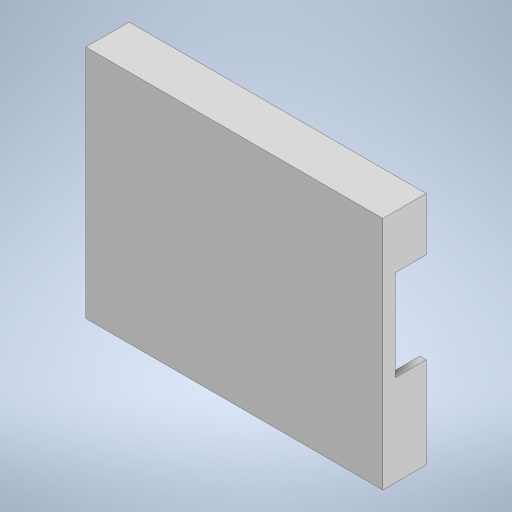
# Autodesk Inventor part: couvercle
Saved by Autodesk Inventor 2024 (Build 280153000, 153)
## iProperties
Created: 2024-03-05
Part Number: couvercle
Material: Générique
Document SubType Name: Modeling
Designer: phaly
Density: 1 g/cm^3
Appearance: Par défaut
Author: phaly
Autodesk Inventor part; units mm, degrees
ref_plane "YZ Plane" through (0, 0, 0) normal (1, 0, 0) x (0, 1, 0)
ref_plane "XZ Plane" through (0, 0, 0) normal (0, 1, 0) x (-1, 0, 0)
sketch "Esquisse1" plane through (0, 0, 0) normal (0, 0, 1) x (1, 0, 0)
  line L0 (-45.5759, 93.3928) -> (-189.5759, 93.3928) projected
  line L1 (-189.5759, 93.3928) -> (-189.5759, -20.6072) projected
  line L2 (-45.5759, -20.6072) -> (-45.5759, 93.3928) projected
  line L3 (-189.5759, -20.6072) -> (-45.5759, -20.6072) projected
  line L4 (-189.5759, 93.3928) -> (-45.5759, 93.3928)
  line L5 (-45.5759, 93.3928) -> (-45.5759, -20.6072)
  line L6 (-45.5759, -20.6072) -> (-189.5759, -20.6072)
  line L7 (-189.5759, -20.6072) -> (-189.5759, 93.3928)
  point P0 (0, 0)
  dimension "d20" = 114
  dimension "d21" = 144
  constraints: 8 end point, 2 parallel, 1 horizontal, 1 perpendicular
  measures "d20" distance of L0.end L1.end
  measures "d21" distance of L1.end L2.start
extrude "Extrusion1" add sketch "Esquisse1" along normal blind 21
sketch "Esquisse2" plane through (0, 0, 0) normal (0, 0, -1) x (-1, 0, 0)
  line L0 (186.5759, -17.6072) -> (48.5759, -17.6072)
  line L1 (48.5759, -17.6072) -> (48.5759, 90.3928)
  line L2 (48.5759, 90.3928) -> (186.5759, 90.3928)
  line L3 (186.5759, 90.3928) -> (186.5759, -17.6072)
  line L4 (189.5759, -20.6072) -> (45.5759, -20.6072) projected
  line L5 (45.5759, 93.3928) -> (189.5759, 93.3928) projected
  line L6 (189.5759, 93.3928) -> (189.5759, -20.6072) projected
  line L7 (45.5759, -20.6072) -> (45.5759, 93.3928) projected
  point P0 (0, 0)
  dimension "d2" = 3
  dimension "d4" = 3
  dimension "d5" = 3
  dimension "d6" = 3
  constraints: 8 end point, 2 parallel, 1 horizontal, 1 perpendicular
  measures "d2" distance between parallel lines of L4 L0
  measures "d4" distance between parallel lines of L6 L3
  measures "d5" distance between parallel lines of L5 L2
  measures "d6" distance between parallel lines of L7 L1
extrude "Extrusion3" cut sketch "Esquisse2" against normal blind 17 contours L0 L1 L2 L3
ref_plane "Plan de construction1" through (-50.5759, 25.8928, -3.5) normal (-1, 0, 0) x (0, 0, 1)
sketch "Esquisse5" plane through (-45.5759, -20.6072, 21) normal (1, 0, 0) x (0, 0, -1)
  line L0 (21, 88.25) -> (6, 88.25)
  line L1 (6, 88.25) -> (6, 44.25)
  line L2 (6, 44.25) -> (21, 44.25)
  line L3 (21, 44.25) -> (21, 88.25)
  line L4 (21, 0) -> (21, 114) projected
  line L5 (21, 0) -> (0, 0) projected
  point P0 (21, 20.6072)
  point P1 (21, 47.25)
  point P2 (13.5, 44.25)
  dimension "d23" = 15
  dimension "d24" = 44.25
  dimension "d25" = 44
  constraints: 8 end point, 2 parallel, 1 collinear, 1 horizontal, 1 midpoint, 1 perpendicular
  measures "d23" distance of L1.end L2.end
  measures "d24" distance from line of L5 L1.end
  measures "d25" distance from line of point (13.5, 44.25) L0
extrude "Extrusion5" cut sketch "Esquisse5" against normal up to surface (3 mm away)
equation "\"d4\" = d2"
equation "\"d5\" = d2"
equation "\"d6\" = d4"
